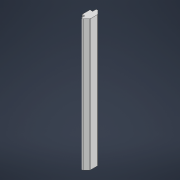
# Autodesk Inventor part: Extrusion_Inside
Saved by Autodesk Inventor 2022.1 (Build 261234000, 234)
## iProperties
Created: 2021-10-12
Part Number: Extrusion_Inside
Material: Generisch
Document SubType Name: Modeling
Designer: Rama
Density: 1 g/cm^3
Appearance: Vorgabe
Author: Rama
Autodesk Inventor part; units mm, degrees
ref_plane "YZ Plane" through (0, 0, 0) normal (1, 0, 0) x (0, 1, 0)
ref_plane "XZ Plane" through (0, 0, 0) normal (0, 1, 0) x (-1, 0, 0)
ref_plane "XY Plane" through (0, 0, 0) normal (0, 0, 1) x (1, 0, 0)
sketch "Skizze1" plane through (0, 0, 0) normal (0, 1, 0) x (-1, 0, 0)
  line L0 (2, 6) -> (-2, 6)
  line L1 (-2, 6) -> (-2, -6)
  line L2 (-2, -6) -> (2, -6)
  line L3 (2, -6) -> (2, 6)
  line L4 (2, 6) -> (-2, -6) construction
  line L5 (-2, 6) -> (2, -6) construction
  line L6 (2, 3) -> (-2, 3)
  line L7 (-2, 3) -> (-2, -3)
  line L8 (-2, -3) -> (2, -3)
  line L9 (2, -3) -> (2, 3)
  line L10 (2, 3) -> (-2, -3) construction
  line L11 (-2, 3) -> (2, -3) construction
  line L12 (-2, 3) -> (1, 6)
  line L13 (-2, 3) -> (2.2426, 3) construction
  line L14 (-2, -3) -> (1, -6)
  line L15 (-2, -3) -> (2.2426, -3) construction
  line L16 (0, 3) -> (4, 3)
  line L17 (4, 3) -> (4, -3)
  line L18 (4, -3) -> (0, -3)
  line L19 (0, -3) -> (0, 3)
  line L20 (0, 3) -> (4, -3) construction
  line L21 (4, 3) -> (0, -3) construction
  point P0 (0, 0)
  point P1 (2, 0)
  dimension "d0" = 4
  dimension "d1" = 12
  dimension "d2" = 6
  dimension "d3" = 45
  dimension "d4" = 45
  dimension "d5" = 4
  dimension "d6" = 6
  constraints: 44 end point, 7 midpoint, 6 parallel, 5 horizontal, 3 perpendicular, 3 point on line, 2 equal length
  measures "d0" distance of L2.end L1.end
  measures "d1" distance of L1.end L0.end
  measures "d2" distance of L7.end L6.end
  measures "d3" angle of L13 L12
  measures "d4" angle of L14 L15
  measures "d5" distance of L17.end L18.end
  measures "d6" distance of L16.end L17.end
extrude "Extrusion1" add sketch "Skizze1" along normal blind 100 contours L3 L6 L12 L0 | L16 L17 L18 L3 | L3 L8 L19 L6 | L6 L19 L8 L1 | L3 L2 L14 L8
sketch "Skizze2" plane through (-4, 0, -3) normal (-1, 0, 0) x (0, 0, 1)
  line L0 (6, 100) -> (0, 100) projected
  line L1 (3, 100) -> (3, 75)
  line L2 (6, 0) -> (6, 100) projected
  line L3 (3, 100) -> (28, 100) construction
  line L4 (3, 75) -> (3, 25)
  point P0 (3, 0)
  dimension "d9" = 25
  dimension "d10" = 90
  dimension "d11" = 50
  dimension "d12" = 180
  constraints: 6 end point, 1 collinear, 1 horizontal, 1 midpoint, 1 parallel, 1 perpendicular
  measures "d9" distance of L1.start L1.end
  measures "d10" angle of L1 L3
  measures "d11" distance of L1.end L4.end
  measures "d12" angle of L4 L1
hole "Bohrung1" at (-4, 75, 0) at (-4, 25, 0) direction (1, 0, 0) diameter 6.1 depth 3.4
fillet "Rundung1" radius 0.4 8 edges at (-3, 75.55, 3) (-3, 74.45, 3) (-3, 74.45, -3) (-3, 75.55, -3) (-3, 24.45, 3) (-3, 25.55, 3) (-3, 24.45, -3) (-3, 25.55, -3)
chamfer "Fase1" distance 0.4 angle 45 2 edges at (2, 50, 3) (2, 50, -3)
fillet "Rundung2" radius 0.8 4 edges at (-1, 50, 6) (-2, 50, 6) (-1, 50, -6) (-2, 50, -6)
